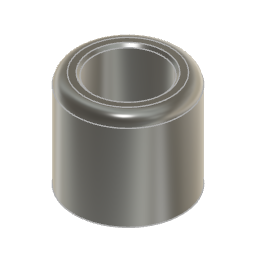
_20mm Dowel Hat, 1_2 dowel.e54efade-bfc4-4de0-bb76-3a28aaa5ddca (Autodesk Fusion 360 design; units mm, degrees)
Autodesk Fusion 360 part; units mm, degrees
sketch "Sketch1" plane through (0, 0, 0) normal (0, 1, 0) x (1, 0, 0)
  line L0 (0, 0) -> (10, 0)
  line L1 (10, 0) -> (10, -3)
  line L2 (10, -3) -> (0, -3)
  line L3 (0, -3) -> (0, 0)
  line L4 (0, -3) -> (6.35, -3)
  line L5 (10, -3) -> (6.35, -3)
  line L6 (6.35, -3) -> (10, -3)
  line L7 (10, -3) -> (10, -18)
  line L8 (10, -18) -> (6.35, -18)
  line L9 (6.35, -18) -> (6.35, -3)
  dimension "d1" = 10
  dimension "d2" = 3
  dimension "d3" = 6.35
  dimension "d5" = 15
  constraint horizontal L0
  constraint vertical L1
  constraint horizontal L2
  constraint vertical L3
  constraint coincident L0.start L3.end
  constraint horizontal L4
  constraint horizontal L5
  constraint horizontal L6
  constraint vertical L7
  constraint horizontal L8
  constraint vertical L9
  measures "d1" distance of L0.start L0.end
  measures "d2" distance of L0.start L2.end
  measures "d3" distance of L2.end L4.end
  measures "d5" distance of L4.end L8.end
revolve "Revolve1" add sketch "Sketch1" angle 360 about axis through (0, 0, 3) along (0, 0, -1)
fillet "Fillet1" radius 2 1 edges at (-9.3233, -3.6162, 18)
chamfer "Chamfer1" distance 0.5 angle 45 1 edges at (-5.9203, -2.2963, 18)
